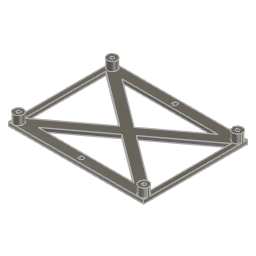
Mainboard Mount (Autodesk Fusion 360 design; units mm, degrees)
Autodesk Fusion 360 part; units mm, degrees
sketch "Sketch1" plane through (0, 0, 0) normal (0, 0, 1) x (1, 0, 0)
  line L0 (50.925, -38.05) -> (-50.925, -38.05) construction
  line L1 (-50.925, -38.05) -> (-50.925, 38.05) construction
  line L2 (-50.925, 38.05) -> (50.925, 38.05) construction
  line L3 (50.925, 38.05) -> (50.925, -38.05) construction
  line L4 (50.925, -38.05) -> (-50.925, 38.05) construction
  line L5 (-50.925, -38.05) -> (50.925, 38.05) construction
  circle A0 centre (-50.925, 38.05) radius 1.4
  circle A1 centre (50.925, 38.05) radius 1.4
  circle A2 centre (-50.925, -38.05) radius 1.4
  circle A3 centre (50.925, -38.05) radius 1.4
  line L6 (54.835, -42.15) -> (-54.835, -42.15)
  line L7 (-54.835, -42.15) -> (-54.835, 42.15)
  line L8 (-54.835, 42.15) -> (54.835, 42.15)
  line L9 (54.835, 42.15) -> (54.835, -42.15)
  line L10 (54.835, -42.15) -> (-54.835, 42.15) construction
  line L11 (-54.835, -42.15) -> (54.835, 42.15) construction
  circle A4 centre (-50.925, 38.05) radius 4
  circle A5 centre (-50.925, -38.05) radius 4
  circle A6 centre (50.925, -38.05) radius 4
  circle A7 centre (50.925, 38.05) radius 4
  line L12 (-50.925, 34.05) -> (50.925, 34.05)
  line L13 (50.925, 34.05) -> (50.925, -34.05)
  line L14 (50.925, -34.05) -> (-50.925, -34.05)
  line L15 (-50.925, -34.05) -> (-50.925, 34.05)
  line L16 (-50.925, 34.05) -> (50.925, -34.05) construction
  line L17 (50.925, 34.05) -> (-50.925, -34.05) construction
  line L18 (53.3192, 34.8457) -> (-48.5308, -41.2543)
  line L19 (48.5308, 41.2543) -> (-53.3192, -34.8457)
  line L20 (53.3192, -34.8457) -> (-48.5308, 41.2543)
  line L21 (-53.6868, 35.1565) -> (48.5301, -41.2538)
  circle A8 centre (0, 38.05) radius 1.75
  circle A9 centre (0, -38.05) radius 1.75
  dimension "d1" = 76.1
  dimension "d2" = 101.85
  dimension "d3" = 2.8
  dimension "d4" = 2.8
  dimension "d5" = 2.8
  dimension "d6" = 2.8
  dimension "d7" = 109.67
  dimension "d8" = 84.3
  dimension "d9" = 8
  dimension "d10" = 8
  dimension "d11" = 8
  dimension "d12" = 8
  dimension "d17" = 3.5
  dimension "d18" = 3.5
  constraint perpendicular L0 L1
  constraint parallel L0 L2
  constraint parallel L1 L3
  constraint horizontal L0
  constraint coincident L4 origin
  constraint coincident L5 origin
  constraint coincident L1.end L2.start
  constraint coincident L2.end L3.start
  constraint coincident L0.end L1.start
  constraint coincident L0.start L3.end
  constraint perpendicular L6 L7
  constraint parallel L6 L8
  constraint parallel L7 L9
  constraint horizontal L6
  constraint coincident L10 origin
  constraint coincident L11 origin
  constraint concentric A3 A6
  constraint perpendicular L12 L13
  constraint parallel L12 L14
  constraint parallel L13 L15
  constraint horizontal L12
  constraint coincident L1 L12.start
  constraint coincident A4 L12.start
  constraint coincident L16 origin
  constraint coincident L17 origin
  constraint coincident A7 L18.start
  constraint coincident A5 L18.end
  constraint tangent A5 L18
  constraint coincident A7 L19.start
  constraint coincident A5 L19.end
  constraint tangent A5 L19
  constraint coincident A6 L20.start
  constraint coincident A4 L20.end
  constraint tangent A4 L20
  constraint coincident A4 L21.start
  constraint coincident A6 L21.end
  constraint tangent A6 L21
  constraint midpoint L2 A8.centre
  constraint midpoint L0 A9.centre
  measures "d1" distance of L0.end L1.end
  measures "d2" distance of L1.end L2.end
  measures "d3" diameter of A0
  measures "d4" diameter of A1
  measures "d5" diameter of A2
  measures "d6" diameter of A3
  measures "d7" distance of L7.end L8.end
  measures "d8" distance of L6.end L7.end
  measures "d9" diameter of A4
  measures "d10" diameter of A5
  measures "d11" diameter of A6
  measures "d12" diameter of A7
  measures "d17" diameter of A8
  measures "d18" diameter of A9
extrude "Extrude1" add sketch "Sketch1" along normal blind 3 contours L6 L7 L9 A5 A6 L14 L18 L21 | L9 A6 | L7 A5 | L9 A6 A7 L13 L18 L20 | A6 L14 L21 | L7 A4 A5 L15 L19 L21 | A5 L14 L18 | L9 A7 | A6 L13 L20 | L13 L14 L18 L20 L21 | L7 A4 L21 | A5 L15 L19 | L14 L15 L18 L19 L21 | L7 L8 L9 A4 A7 L12 L19 L20 | A7 L13 L18 | L18 L19 L20 L21 | A4 L21 | A7 L12 L19 | L12 L13 L18 L19 L20 | L12 L15 L19 L20 L21 | A4 L12 L20 | A4 L15 L21 | A8 | A9 picked at (53.9983, -38.05) picked at (-53.9983, -38.05) picked at (53.9983, 38.05)
extrude "Extrude2" add sketch "Sketch1" along normal blind 10 contours L9 A6 | L7 A5 | L9 A7 | L7 A4 L21 | A4 L21 picked at (53.9983, -38.05) picked at (-53.9983, -38.05) picked at (53.9983, 38.05)
extrude "Extrude3" cut sketch "Sketch1" along normal blind 7 contours A8 | A9
